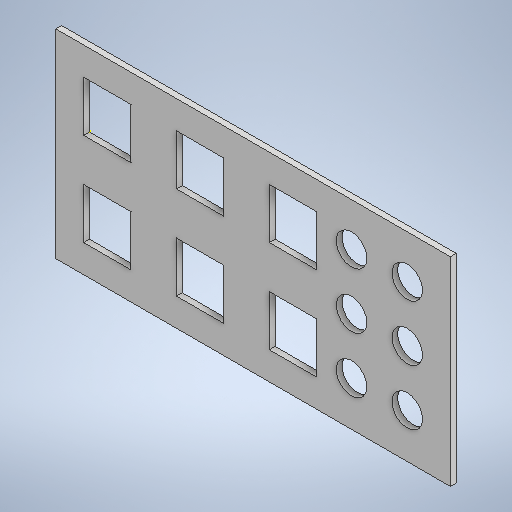
# Autodesk Inventor part: faceplate
Saved by Autodesk Inventor 2025 (Build 290162000, 162)
## iProperties
Created: 2024-08-10
Part Number: faceplate
Material: Generic
Document SubType Name: Modeling
Designer: ethan
Density: 1 g/cm^3
Appearance: Default
Author: ethan
Autodesk Inventor part; units mm, degrees
ref_plane "YZ Plane" through (0, 0, 0) normal (1, 0, 0) x (0, 1, 0)
ref_plane "XZ Plane" through (0, 0, 0) normal (0, 1, 0) x (-1, 0, 0)
ref_plane "XY Plane" through (0, 0, 0) normal (0, 0, 1) x (1, 0, 0)
sketch "Sketch1" plane through (0, 0, 0) normal (0, 0, 1) x (1, 0, 0)
  point P0 (0, 0)
sketch "Sketch2" plane through (0, 0, 0) normal (0, 0, 1) x (1, 0, 0)
  line L0 (0, 0) -> (20.4, 0)
  line L1 (20.4, 0) -> (20.4, 21.7)
  line L2 (20.4, 21.7) -> (0, 21.7)
  line L3 (0, 21.7) -> (0, 0)
  line L4 (40, 0) -> (60.4, 0)
  line L5 (60.4, 0) -> (60.4, 21.7)
  line L6 (60.4, 21.7) -> (40, 21.7)
  line L7 (40, 21.7) -> (40, 0)
  line L8 (80, 0) -> (100.4, 0)
  line L9 (100.4, 0) -> (100.4, 21.7)
  line L10 (100.4, 21.7) -> (80, 21.7)
  line L11 (80, 21.7) -> (80, 0)
  line L12 (0, -40) -> (20.4, -40)
  line L13 (20.4, -40) -> (20.4, -18.3)
  line L14 (20.4, -18.3) -> (0, -18.3)
  line L15 (0, -18.3) -> (0, -40)
  line L16 (40, -40) -> (60.4, -40)
  line L17 (60.4, -40) -> (60.4, -18.3)
  line L18 (60.4, -18.3) -> (40, -18.3)
  line L19 (40, -18.3) -> (40, -40)
  line L20 (80, -40) -> (100.4, -40)
  line L21 (100.4, -40) -> (100.4, -18.3)
  line L22 (100.4, -18.3) -> (80, -18.3)
  line L23 (80, -18.3) -> (80, -40)
  line L24 (100.4, 21.7) -> (175.4, 21.7) construction
  line L25 (175.4, 21.7) -> (175.4, -53.3) construction
  line L26 (175.4, -53.3) -> (100.4, -53.3) construction
  line L27 (100.4, -53.3) -> (100.4, 21.7) construction
  circle A0 centre (115.4, 15.1) radius 6.6 construction
  line L28 (115.4, 15.1) -> (115.4, -53.3) construction
  circle A1 centre (115.4, -8.9) radius 6.6 construction
  circle A2 centre (115.4, -32.9) radius 6.6 construction
  line L29 (100.4, 15.1) -> (200.3961, 15.1) construction
  circle A3 centre (139.4, 15.1) radius 6.6 construction
  circle A4 centre (139.4, -8.9) radius 6.6 construction
  circle A5 centre (139.4, -32.9) radius 6.6 construction
  circle A6 centre (115.4, 15.1) radius 6.6
  circle A7 centre (139.4, 15.1) radius 6.6 construction
  circle A8 centre (139.4, 15.1) radius 6.6
  circle A9 centre (115.4, -8.9) radius 6.6 construction
  circle A10 centre (115.4, -8.9) radius 6.6
  circle A11 centre (139.4, -8.9) radius 6.6 construction
  circle A12 centre (139.4, -8.9) radius 6.6
  circle A13 centre (115.4, -32.9) radius 6.6 construction
  circle A14 centre (115.4, -32.9) radius 6.6
  circle A15 centre (139.4, -32.9) radius 6.6 construction
  circle A16 centre (139.4, -32.9) radius 6.6
  line L30 (0, 21.7) -> (-12, 21.7) construction
  line L31 (-12, 21.7) -> (-12, 33.7) construction
  line L32 (-12, 33.7) -> (0, 33.7) construction
  line L33 (0, 33.7) -> (0, 21.7) construction
  line L34 (146, -40) -> (158, -40) construction
  line L35 (158, -40) -> (158, -52) construction
  line L36 (158, -52) -> (146, -52) construction
  line L37 (146, -52) -> (146, -40) construction
  line L38 (139.4, -32.9) -> (139.4, -74.4589) construction
  line L39 (-12, 33.7) -> (158, 33.7)
  line L40 (158, 33.7) -> (158, -52)
  line L41 (158, -52) -> (-12, -52)
  line L42 (-12, -52) -> (-12, 33.7)
  point P0 (146, -46)
  dimension "d0" = 20.4
  dimension "d1" = 21.7
  dimension "d5" = 40
  dimension "d8" = 40
  dimension "d11" = 75
  dimension "d12" = 75
  dimension "d13" = 13.2
  dimension "d14" = 15
  dimension "d15" = 13.2
  dimension "d16" = 24
  dimension "d17" = 13.2
  dimension "d18" = 24
  dimension "d19" = 61.7
  dimension "d20" = 13.2
  dimension "d21" = 24
  dimension "d22" = 13.2
  dimension "d23" = 13.2
  dimension "d26" = 24
  dimension "d29" = 24
  dimension "d32" = 12
  dimension "d33" = 12
  dimension "d34" = 12
  dimension "d35" = 12
  dimension "d36" = 6.6
  constraints: 86 end point, 17 centre point, 8 horizontal, 8 parallel, 7 perpendicular, 6 coincident, 5 point on line, 3 collinear, 3 vertical, 1 midpoint, 1 tangent, 58 other
  measures "d0" distance of L2.end L1.end
  measures "d1" distance of L0.end L1.end
  measures "d5" distance of L1.end L5.end
  measures "d8" distance of L1.end L13.end
  measures "d11" distance of L9.end L24.end
  measures "d12" distance of L24.end L25.end
  measures "d13" diameter of A0
  measures "d14" distance from line of L9 L28.start
  measures "d15" diameter of A1
  measures "d16" distance of A1.centre L28.start
  measures "d17" diameter of A2
  measures "d18" distance of A1.centre A2.centre
  measures "d19" distance between parallel lines of L20 L10
  measures "d20" diameter of A3
  measures "d21" distance of A3.centre L28.start
  measures "d22" diameter of A4
  measures "d23" diameter of A5
  measures "d26" distance of L28.start A7.centre
  measures "d29" distance of L28.start A9.centre
  measures "d32" distance of L31.end L32.end
  measures "d33" distance of L30.end L31.end
  measures "d34" distance of L35.end L36.end
  measures "d35" distance of L34.end L35.end
  measures "d36" distance from line of point (146, -46) L38
extrude "Extrusion1" add sketch "Sketch2" along normal blind 2.5
body "Solid1"
